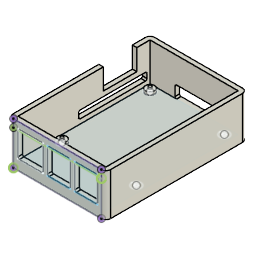
Case (Autodesk Fusion 360 design; units mm, degrees)
part number: 2026-04-01-16-26-12-971
Autodesk Fusion 360 part; units mm, degrees
sketch "Sketch1" plane through (0, 0, 0) normal (0, 0, 1) x (1, 0, 0)
  line L0 (3, 0) -> (61, 0)
  line L1 (64, 3) -> (64, 90)
  line L2 (61, 93) -> (3, 93)
  line L3 (0, 90) -> (0, 3)
  arc A0 (3, 93) -> (0, 90) centre (3, 90) ccw
  arc A1 (64, 90) -> (61, 93) centre (61, 90) ccw
  arc A2 (61, 0) -> (64, 3) centre (61, 3) ccw
  arc A3 (0, 3) -> (3, 0) centre (3, 3) ccw
  point P0 (64, 0)
  point P1 (0, 93)
  dimension "d1" = 64
  dimension "d2" = 93
  dimension "d3" = 3
  dimension "d4" = 3
  constraint horizontal L0
  constraint vertical L1
  constraint horizontal L2
  constraint vertical L3
  constraint coincident P1 L2
  constraint coincident P1 L3
  constraint tangent L2 A0
  constraint tangent L3 A0
  constraint tangent L1 A1
  constraint tangent L2 A1
  constraint equal A0 A1
  constraint coincident P0 L0
  constraint coincident P0 L1
  constraint tangent L0 A2
  constraint tangent L1 A2
  constraint equal A0 A2
  constraint coincident origin L0
  constraint coincident origin L3
  constraint tangent L0 A3
  constraint tangent L3 A3
  measures "d1" distance of origin P0
  measures "d2" distance of origin P1
  measures "d3" radius of A0
  measures "d4" radius of A3
extrude "Extrude1" add sketch "Sketch1" along normal blind 3
sketch "Sketch4" plane through (0, 0, 3) normal (0, 0, 1) x (-1, 0, 0)
  arc A0 (0, -3) -> (-3, 0) centre (-3, -3) ccw
  line L0 (-3, 0) -> (-61, 0)
  arc A1 (-61, 0) -> (-64, -3) centre (-61, -3) ccw
  line L1 (-64, -3) -> (-64, -90)
  arc A2 (-64, -90) -> (-61, -93) centre (-61, -90) ccw
  line L2 (-61, -93) -> (-3, -93)
  arc A3 (-3, -93) -> (0, -90) centre (-3, -90) ccw
  line L3 (0, -90) -> (0, -3)
  line L4 (-3, -3) -> (-61, -3)
  line L5 (-61, -3) -> (-61, -90)
  line L6 (-61, -90) -> (-3, -90)
  line L7 (-3, -90) -> (-3, -3)
  dimension "d11" = 58
  dimension "d12" = 87
  dimension "d13" = 3
  dimension "d14" = 3
  constraint horizontal L4
  constraint vertical L5
  constraint horizontal L6
  constraint vertical L7
  measures "d11" distance of A0.centre A1.centre
  measures "d12" distance of A0.centre A3.centre
  measures "d13" distance of L3 L7
  measures "d14" distance of L0 L4
extrude "Extrude2" add sketch "Sketch4" along normal blind 25
sketch "Sketch5" plane through (0, 0, 0) normal (0, -1, 0) x (1, 0, 0)
  line L0 (3, 0) -> (61, 0)
  line L1 (61, 0) -> (61, 23)
  line L2 (3, 23) -> (61, 23)
  line L3 (6, 6.8) -> (22.5, 6.8)
  line L4 (22.5, 6.8) -> (22.5, 23.8)
  line L5 (22.5, 23.8) -> (6, 23.8)
  line L6 (6, 23.8) -> (6, 6.8)
  line L7 (3, 0) -> (3, 23)
  line L8 (25.5, 23.8) -> (40.45, 23.8)
  line L9 (40.45, 23.8) -> (40.45, 6.8)
  line L10 (40.45, 6.8) -> (25.5, 6.8)
  line L11 (25.5, 6.8) -> (25.5, 23.8)
  line L12 (43.45, 6.8) -> (58.4, 6.8)
  line L13 (58.4, 6.8) -> (58.4, 23.8)
  line L14 (58.4, 23.8) -> (43.45, 23.8)
  line L15 (43.45, 23.8) -> (43.45, 6.8)
  line L16 (3, 0) -> (61, 0)
  line L17 (61, 0) -> (61, 28)
  line L18 (61, 28) -> (3, 28)
  line L19 (3, 28) -> (3, 0)
  dimension "d21" = 16.5
  dimension "d22" = 17
  dimension "d23" = 3
  dimension "d26" = 14.95
  dimension "d27" = 17
  dimension "d29" = 14.95
  dimension "d30" = 17
  dimension "d31" = 3
  dimension "d34" = 3
  dimension "d45" = 6.8
  constraint horizontal L3
  constraint vertical L4
  constraint horizontal L5
  constraint vertical L6
  constraint horizontal L8
  constraint vertical L9
  constraint horizontal L10
  constraint vertical L11
  constraint horizontal L12
  constraint vertical L13
  constraint horizontal L14
  constraint vertical L15
  measures "d21" distance of L3.start L3.end
  measures "d22" distance of L3.start L5.end
  measures "d23" distance of L6 L7
  measures "d26" distance of L8.start L8.end
  measures "d27" distance of L8.start L10.end
  measures "d29" distance of L12.start L12.end
  measures "d30" distance of L12.start L14.end
  measures "d31" distance of L9 L15
  measures "d34" distance of L4 L11
  measures "d45" distance of L0 L3
extrude "Extrude4" cut sketch "Sketch5" against normal blind 3 contours L2 L4 L5 L6 | L2 L3 L4 L6 | L2 L12 L13 L15 | L2 L13 L14 L15 | L2 L8 L9 L11 | L2 L9 L10 L11
sketch "Sketch6" plane through (0, 0, 3) normal (0, 0, 1) x (-1, 0, 0)
  line L0 (-3, -3) -> (-61, -3)
  line L1 (-61, -3) -> (-61, -90)
  line L2 (-61, -90) -> (-3, -90)
  line L3 (-3, -90) -> (-3, -3)
  circle A0 centre (-7.5, -85.5) radius 1
  circle A1 centre (-7.5, -85.5) radius 3
  circle A2 centre (-56.5, -85.5) radius 1
  circle A3 centre (-56.5, -85.5) radius 3
  circle A4 centre (-56.5, -27.5) radius 1
  circle A5 centre (-56.5, -27.5) radius 3
  circle A6 centre (-7.5, -27.5) radius 1
  circle A7 centre (-7.5, -27.5) radius 3
  dimension "d35" = 2
  dimension "d36" = 4.5
  dimension "d37" = 4.5
  dimension "d38" = 6
  dimension "d59" = 2
  dimension "d60" = 4.5
  dimension "d61" = 4.5
  dimension "d62" = 6
  dimension "d63" = 2
  dimension "d64" = 4.5
  dimension "d65" = 58
  dimension "d66" = 6
  dimension "d67" = 2
  dimension "d68" = 4.5
  dimension "d69" = 58
  dimension "d70" = 6
  constraint concentric A0 A1
  constraint concentric A2 A3
  constraint concentric A4 A5
  constraint concentric A6 A7
  measures "d35" diameter of A0
  measures "d36" distance of L2 A0.centre
  measures "d37" distance of L3 A0.centre
  measures "d38" diameter of A1
  measures "d59" diameter of A2
  measures "d60" distance of L2 A2.centre
  measures "d61" distance of L1 A2.centre
  measures "d62" diameter of A3
  measures "d63" diameter of A4
  measures "d64" distance of L1 A4.centre
  measures "d65" distance of A2.centre A4.centre
  measures "d66" diameter of A5
  measures "d67" diameter of A6
  measures "d68" distance of L3 A6.centre
  measures "d69" distance of A0.centre A6.centre
  measures "d70" diameter of A7
extrude "Extrude6" cut sketch "Sketch6" against normal blind 3 contours A0 | A2 | A4 | A6
extrude "Extrude7" add sketch "Sketch6" along normal blind 0.5 contours A1
sketch "Sketch7" plane through (0, 0, 0) normal (-1, 0, 0) x (0, -1, 0)
  line L0 (-90, 0) -> (-3, 0)
  line L1 (-3, 0) -> (-3, 28)
  line L2 (-3, 28) -> (-90, 28)
  line L3 (-90, 28) -> (-90, 0)
  line L4 (-88, 6) -> (-43, 6)
  line L5 (-43, 6) -> (-43, 11)
  line L6 (-43, 11) -> (-88, 11)
  line L7 (-88, 11) -> (-88, 6)
  dimension "d46" = 45
  dimension "d47" = 5
  dimension "d50" = 6
  constraint horizontal L4
  constraint vertical L5
  constraint horizontal L6
  constraint vertical L7
  measures "d46" distance of L4.start L4.end
  measures "d47" distance of L4.start L6.end
  measures "d50" distance of L0 L4
extrude "Extrude8" cut sketch "Sketch7" against normal blind 3 contours L4 L5 L6 L7
sketch "Sketch8" plane through (0, 93, 0) normal (0, 1, 0) x (-1, 0, 0)
  line L0 (-61, 0) -> (-3, 0)
  line L1 (-3, 0) -> (-3, 28)
  line L2 (-3, 28) -> (-61, 28)
  line L3 (-61, 28) -> (-61, 0)
  line L4 (-44.5, 3) -> (-19.5, 3)
  line L5 (-19.5, 3) -> (-19.5, 11)
  line L6 (-19.5, 11) -> (-44.5, 11)
  line L7 (-44.5, 11) -> (-44.5, 3)
  line L8 (-3, 0) -> (-3, 23)
  line L9 (-3, 0) -> (-61, 0)
  dimension "d51" = 25
  dimension "d52" = 8
  dimension "d53" = 16.5
  dimension "d54" = 3
  constraint horizontal L4
  constraint vertical L5
  constraint horizontal L6
  constraint vertical L7
  measures "d51" distance of L4.start L4.end
  measures "d52" distance of L4.start L6.end
  measures "d53" distance of L5 L8
  measures "d54" distance of L4 L9
extrude "Extrude9" cut sketch "Sketch8" against normal blind 3 contours L4 L5 L6 L7
extrude "Extrude10" add 1 faces at (9.6751, 86.3269, 3.5) along direction (0, 0, 1) blind 1.5
extrude "Extrude11" add sketch "Sketch6" along normal blind 2 contours A3 | A5 | A7
extrude "Extrude13" add sketch "Sketch6" along normal blind 3 contours A4
extrude "Extrude14" add sketch "Sketch6" along normal blind 3 contours A0 | A2 | A6
sketch "Sketch11" plane through (0, 0, 0) normal (-1, 0, 0) x (0, -1, 0)
  line L0 (-43, 6) -> (-88, 6)
  line L1 (-88, 6) -> (-88, 11)
  line L2 (-88, 11) -> (-43, 11)
  line L3 (-43, 11) -> (-43, 6)
  line L4 (-90, 0) -> (-3, 0)
  line L5 (-3, 0) -> (-3, 28)
  line L6 (-3, 28) -> (-90, 28)
  line L7 (-90, 28) -> (-90, 0)
  line L8 (-81.3, 28) -> (-59.3, 28)
  line L9 (-59.3, 28) -> (-59.3, 14.2)
  line L10 (-59.3, 14.2) -> (-81.3, 14.2)
  line L11 (-81.3, 14.2) -> (-81.3, 28)
  dimension "d85" = 22
  dimension "d86" = 13.8
  dimension "d87" = 8.7
  constraint horizontal L8
  constraint vertical L9
  constraint horizontal L10
  constraint vertical L11
  constraint coincident L6 L8.start
  measures "d85" distance of L8.start L8.end
  measures "d86" distance of L8.start L10.end
  measures "d87" distance of L7 L11
extrude "Extrude15" cut sketch "Sketch11" against normal blind 3 contours L6 L8 L9 L10 L11
fillet "Fillet1" radius 1 1 edges at (1.5, 81.3, 14.2)
fillet "Fillet2" radius 1 21 edges at (1.5, 59.3, 14.2) (44.5, 91.5, 3) (44.5, 91.5, 11) (19.5, 91.5, 3) (19.5, 91.5, 11) (1.5, 43, 6) (6, 1.5, 6.8) (25.5, 1.5, 6.8) (43.45, 1.5, 6.8) (6, 1.5, 23.8) (25.5, 1.5, 23.8) (43.45, 1.5, 23.8) (40.45, 1.5, 23.8) (22.5, 1.5, 23.8) (58.4, 1.5, 23.8) (1.5, 88, 11) (1.5, 88, 6) (22.5, 1.5, 6.8) (40.45, 1.5, 6.8) (58.4, 1.5, 6.8) (1.5, 43, 11)
delete_face "DeleteFace1" 1 faces at (1, 80.5358, 14.2282)
delete_face "DeleteFace2" 1 faces at (1, 59.4854, 14.6199)
